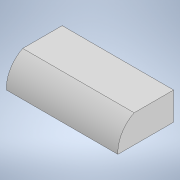
# Autodesk Inventor part: Container
Saved by Autodesk Inventor 2020 (Build 240168000, 168)
## iProperties
Created: 2021-05-03
Part Number: Container
Material: Generic
Document SubType Name: Modeling
Designer: chick
Density: 1 g/cm^3
Appearance: Default
Author: chick
Autodesk Inventor part; units mm, degrees
ref_plane "YZ Plane" through (0, 0, 0) normal (1, 0, 0) x (0, 1, 0)
ref_plane "XZ Plane" through (0, 0, 0) normal (0, 1, 0) x (-1, 0, 0)
ref_plane "XY Plane" through (0, 0, 0) normal (0, 0, 1) x (1, 0, 0)
sketch "Sketch1" plane through (0, 0, 0) normal (1, 0, 0) x (0, 1, 0)
  line L0 (0, 0) -> (0, -100)
  line L1 (0, -100) -> (50, -100)
  line L2 (50, -100) -> (50, -29.2097)
  arc A0 (50, -29.2097) -> (0, 0) centre (2.9206, -52.3995) ccw
  dimension "d0" = 100
  dimension "d1" = 50
  constraints: 6 end point, 2 perpendicular, 2 point on circle, 1 centre point, 1 vertical
  measures "d0" distance of L0.start L0.end
  measures "d1" distance of L0.end L1.end
extrude "Extrusion1" add sketch "Sketch1" against normal blind 200
sketch "Sketch4" plane through (0, 0, -100) normal (0, 0, -1) x (-1, 0, 0)
  line L0 (5, 45) -> (5, 5)
  line L1 (5, 5) -> (195, 5)
  line L2 (195, 5) -> (195, 45)
  line L3 (195, 45) -> (5, 45)
  line L4 (0, 50) -> (200, 50) projected
  line L5 (0, 0) -> (0, 50) projected
  line L6 (200, 50) -> (200, 0) projected
  line L7 (0, 0) -> (200, 0) projected
  dimension "d5" = 5
  dimension "d6" = 5
  dimension "d7" = 5
  dimension "d8" = 5
  constraints: 8 end point, 3 perpendicular, 1 vertical
  measures "d5" distance between parallel lines of L3 L4
  measures "d6" distance between parallel lines of L5 L0
  measures "d7" distance between parallel lines of L6 L2
  measures "d8" distance between parallel lines of L7 L1
extrude "Extrusion2" cut sketch "Sketch4" against normal blind 70 contours L3 L2 L1 L0
sketch "Sketch5" plane through (0, 0, -100) normal (0, -1, 0) x (1, 0, 0)
  circle A0 centre (-10, 90) radius 1.5
  circle A1 centre (-10, 10) radius 1.5
  circle A2 centre (-190, 90) radius 1.5
  circle A3 centre (-190, 10) radius 1.5
  line L0 (0, 100) -> (-200, 100) projected
  line L1 (0, 0) -> (-200, 0) projected
  line L2 (0, 100) -> (0, 0) projected
  line L3 (-200, 0) -> (-200, 100) projected
  point P0 (-195, 0)
  dimension "d11" = 3
  dimension "d12" = 3
  dimension "d13" = 3
  dimension "d14" = 3
  dimension "d15" = 10
  dimension "d16" = 10
  dimension "d17" = 10
  dimension "d18" = 10
  dimension "d19" = 10
  dimension "d20" = 10
  dimension "d22" = 10
  dimension "d23" = 10
  constraints: 4 centre point
  measures "d11" diameter of A0
  measures "d12" diameter of A1
  measures "d13" diameter of A2
  measures "d14" diameter of A3
  measures "d15" distance from line of A0.centre L0
  measures "d16" distance from line of L1 A1.centre
  measures "d17" distance from line of L2 A0.centre
  measures "d18" distance from line of A1.centre L2
  measures "d19" distance from line of L3 A2.centre
  measures "d20" distance from line of L0 A2.centre
  measures "d22" distance from line of L3 A3.centre
  measures "d23" distance from line of L1 A3.centre
extrude "Extrusion3" cut sketch "Sketch5" against normal blind 10 contours A0 | A1 | A2 | A3
equation "\"d1\" = 0.5 * d0"
equation "\"d16\" = d15"
equation "\"d18\" = d17"
equation "\"d19\" = d17"
equation "\"d20\" = d15"
equation "\"d22\" = d17"
equation "\"d23\" = d15"
body "Solid1"
